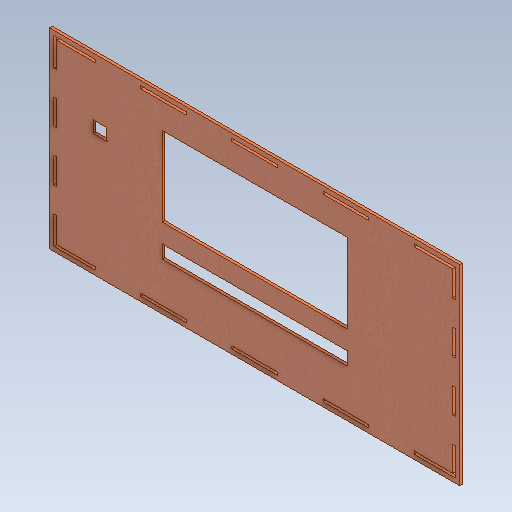
# Autodesk Inventor part: Frontal Arduino
Saved by Autodesk Inventor 2020.3 (Build 243373000, 373)
## iProperties
Created: 2020-05-07
Part Number: Frontal Arduino
Material: Madera (nogal)
Document SubType Name: Modeling
Designer: miosh
Density: 0.55 g/cm^3
Appearance: Nogal - Natural pulido
Author: miosh
Autodesk Inventor part; units mm, degrees
ref_plane "YZ Plane" through (0, 0, 0) normal (1, 0, 0) x (0, 1, 0)
ref_plane "XZ Plane" through (0, 0, 0) normal (0, 1, 0) x (-1, 0, 0)
ref_plane "XY Plane" through (0, 0, 0) normal (0, 0, 1) x (1, 0, 0)
sketch "Boceto1" plane through (0, 0, 0) normal (0, 0, 1) x (1, 0, 0)
  line L0 (0, 0) -> (0, 210)
  line L1 (0, 210) -> (450, 210)
  line L2 (450, 210) -> (450, 0)
  line L3 (450, 0) -> (0, 0)
  line L4 (5, 5) -> (5, 35.71)
  line L5 (5, 5) -> (50, 5)
  line L6 (50, 5) -> (50, 8)
  line L7 (5, 35.71) -> (8, 35.71)
  line L8 (50, 8) -> (8, 8)
  line L9 (8, 8) -> (8, 35.71)
  line L10 (5, 63.43) -> (5, 91.14)
  line L11 (5, 118.86) -> (5, 146.57)
  line L12 (5, 174.29) -> (5, 205)
  line L13 (5, 205) -> (50, 205)
  line L14 (5, 63.43) -> (8, 63.43)
  line L15 (8, 63.43) -> (8, 91.14)
  line L16 (8, 91.14) -> (5, 91.14)
  line L17 (5, 118.86) -> (8, 118.86)
  line L18 (8, 118.86) -> (8, 146.57)
  line L19 (8, 146.57) -> (5, 146.57)
  line L20 (50, 205) -> (50, 202)
  line L21 (5, 174.29) -> (8, 174.29)
  line L22 (8, 174.29) -> (8, 202)
  line L23 (8, 202) -> (50, 202)
  line L24 (100, 205) -> (150, 205)
  line L25 (200, 205) -> (250, 205)
  line L26 (300, 205) -> (350, 205)
  line L27 (400, 205) -> (445, 205)
  line L28 (445, 205) -> (445, 174.29)
  line L29 (100, 205) -> (100, 202)
  line L30 (100, 202) -> (150, 202)
  line L31 (150, 202) -> (150, 205)
  line L32 (200, 205) -> (200, 202)
  line L33 (200, 202) -> (250, 202)
  line L34 (250, 202) -> (250, 205)
  line L35 (300, 205) -> (300, 202)
  line L36 (300, 202) -> (350, 202)
  line L37 (350, 202) -> (350, 205)
  line L38 (400, 205) -> (400, 202)
  line L39 (445, 174.29) -> (442, 174.29)
  line L40 (442, 174.29) -> (442, 202)
  line L41 (442, 202) -> (400, 202)
  line L42 (445, 146.57) -> (445, 118.86)
  line L43 (445, 91.14) -> (445, 63.43)
  line L44 (445, 35.71) -> (445, 5)
  line L45 (445, 5) -> (400, 5)
  line L46 (445, 35.71) -> (442, 35.71)
  line L47 (400, 5) -> (400, 8)
  line L48 (400, 8) -> (442, 8)
  line L49 (442, 8) -> (442, 35.71)
  line L50 (445, 63.43) -> (442, 63.43)
  line L51 (442, 63.43) -> (442, 91.14)
  line L52 (442, 91.14) -> (445, 91.14)
  line L53 (445, 118.86) -> (442, 118.86)
  line L54 (442, 118.86) -> (442, 146.57)
  line L55 (442, 146.57) -> (445, 146.57)
  line L56 (100, 5) -> (150, 5)
  line L57 (200, 5) -> (250, 5)
  line L58 (300, 5) -> (350, 5)
  line L59 (100, 5) -> (100, 8)
  line L60 (100, 8) -> (150, 8)
  line L61 (150, 8) -> (150, 5)
  line L62 (200, 5) -> (200, 8)
  line L63 (200, 8) -> (250, 8)
  line L64 (250, 8) -> (250, 5)
  line L65 (300, 5) -> (300, 8)
  line L66 (300, 8) -> (350, 8)
  line L67 (350, 8) -> (350, 5)
  line L68 (225, 174.29) -> (326.5, 174.29)
  line L69 (225, 174.29) -> (123.5, 174.29)
  line L70 (326.5, 174.29) -> (326.5, 87.29)
  line L71 (326.5, 87.29) -> (123.5, 87.29)
  line L72 (123.5, 87.29) -> (123.5, 174.29)
  line L73 (225, 52) -> (326.5, 52)
  line L74 (225, 52) -> (123.5, 52)
  line L75 (123.5, 52) -> (123.5, 66.5)
  line L76 (123.5, 66.5) -> (326.5, 66.5)
  line L77 (326.5, 66.5) -> (326.5, 52)
  line L78 (48, 146.57) -> (63, 146.57)
  line L79 (63, 146.57) -> (63, 133.57)
  line L80 (63, 133.57) -> (48, 133.57)
  line L81 (48, 133.57) -> (48, 146.57)
  dimension "d0" = 210
  dimension "d1" = 450
  dimension "d2" = 30.71
  dimension "d3" = 45
  dimension "d4" = 3
  dimension "d5" = 3
  dimension "d7" = 27.71
  dimension "d8" = 27.72
  dimension "d9" = 27.71
  dimension "d10" = 27.72
  dimension "d12" = 30.71
  dimension "d13" = 45
  dimension "d14" = 27.72
  dimension "d15" = 3
  dimension "d17" = 3
  dimension "d19" = 3
  dimension "d20" = 3
  dimension "d21" = 50
  dimension "d22" = 50
  dimension "d23" = 50
  dimension "d24" = 50
  dimension "d25" = 50
  dimension "d26" = 50
  dimension "d27" = 50
  dimension "d28" = 45
  dimension "d29" = 30.71
  dimension "d30" = 3
  dimension "d31" = 3
  dimension "d33" = 3
  dimension "d35" = 50
  dimension "d36" = 3
  dimension "d37" = 3
  dimension "d38" = 27.72
  dimension "d39" = 27.71
  dimension "d40" = 27.72
  dimension "d41" = 27.71
  dimension "d42" = 27.72
  dimension "d43" = 30.71
  dimension "d44" = 3
  dimension "d45" = 3
  dimension "d46" = 3
  dimension "d47" = 3
  dimension "d48" = 50
  dimension "d49" = 50
  dimension "d50" = 50
  dimension "d51" = 50
  dimension "d52" = 50
  dimension "d53" = 50
  dimension "d54" = 50
  dimension "d55" = 3
  dimension "d56" = 3
  dimension "d58" = 3
  dimension "d59" = 5
  dimension "d60" = 5
  dimension "d61" = 5
  dimension "d62" = 5
  dimension "d63" = 5
  dimension "d64" = 5
  dimension "d65" = 5
  dimension "d66" = 5
  dimension "d67" = 5
  dimension "d68" = 5
  dimension "d69" = 5
  dimension "d70" = 5
  constraints: 164 end point, 35 perpendicular, 13 horizontal, 11 vertical, 10 point on line, 6 parallel
  measures "d0" distance of L0.start L0.end
  measures "d1" distance of L0.end L1.end
  measures "d2" distance of L4.start L4.end
  measures "d3" distance of L4.start L5.end
  measures "d4" distance of L5.end L6.end
  measures "d5" distance of L4.end L7.end
  measures "d7" distance of L10.start L10.end
  measures "d8" distance of L10.end L11.start
  measures "d9" distance of L11.start L11.end
  measures "d10" distance of L11.end L12.start
  measures "d12" distance of L12.start L12.end
  measures "d13" distance of L12.end L13.end
  measures "d14" distance of L4.end L10.start
  measures "d15" distance of L10.start L14.end
  measures "d17" distance of L11.start L17.end
  measures "d19" distance of L13.end L20.end
  measures "d20" distance of L12.start L21.end
  measures "d21" distance of L13.end L24.start
  measures "d22" distance of L24.start L24.end
  measures "d23" distance of L24.end L25.start
  measures "d24" distance of L25.start L25.end
  measures "d25" distance of L25.end L26.start
  measures "d26" distance of L26.start L26.end
  measures "d27" distance of L26.end L27.start
  measures "d28" distance of L27.start L27.end
  measures "d29" distance of L27.end L28.end
  measures "d30" distance of L24.start L29.end
  measures "d31" distance of L25.start L32.end
  measures "d33" distance of L26.start L35.end
  measures "d35" distance of L35.end L36.end
  measures "d36" distance of L27.start L38.end
  measures "d37" distance of L28.end L39.end
  measures "d38" distance of L28.end L42.start
  measures "d39" distance of L42.start L42.end
  measures "d40" distance of L42.end L43.start
  measures "d41" distance of L43.start L43.end
  measures "d42" distance of L43.end L44.start
  measures "d43" distance of L44.start L44.end
  measures "d44" distance of L44.start L46.end
  measures "d45" distance of L45.end L47.end
  measures "d46" distance of L43.end L50.end
  measures "d47" distance of L42.end L53.end
  measures "d48" distance of L5.end L56.start
  measures "d49" distance of L56.start L56.end
  measures "d50" distance of L56.end L57.start
  measures "d51" distance of L57.start L57.end
  measures "d52" distance of L57.end L58.start
  measures "d53" distance of L58.start L58.end
  measures "d54" distance of L58.end L45.end
  measures "d55" distance of L56.start L59.end
  measures "d56" distance of L57.start L62.end
  measures "d58" distance of L58.start L65.end
  measures "d59" distance between parallel lines of L3 L5
  measures "d60" distance between parallel lines of L3 L56
  measures "d61" distance between parallel lines of L3 L57
  measures "d62" distance between parallel lines of L3 L45
  measures "d63" distance between parallel lines of L24 L1
  measures "d64" distance between parallel lines of L1 L25
  measures "d65" distance between parallel lines of L1 L26
  measures "d66" distance between parallel lines of L1 L27
  measures "d67" distance between parallel lines of L13 L1
  measures "d68" distance between parallel lines of L0 L12
  measures "d69" distance between parallel lines of L0 L11
  measures "d70" distance between parallel lines of L0 L10
extrude "Extrusión1" add sketch "Boceto1" along normal blind 3
